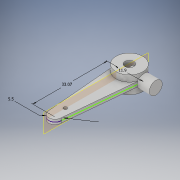
# Autodesk Inventor part: Nose Gear Steering Arm
Saved by Autodesk Inventor 2018 (Build 220112000, 112)
## iProperties
Created: 2018-08-04
Part Number: Nose Gear Steering Arm
Material: Generic
Document SubType Name: Modeling
Designer: Michael Gunderman
Density: 3.52387 g/cm^3
Appearance: Default
Mass: 5 g
Surface Area: 12.8518 cm^2
Volume: 1.41889 cm^3
Author: Michael Gunderman
Autodesk Inventor part; units mm, degrees
ref_plane "YZ Plane" through (0, 0, 0) normal (1, 0, 0) x (0, 1, 0)
ref_plane "XZ Plane" through (0, 0, 0) normal (0, 1, 0) x (-1, 0, 0)
ref_plane "XY Plane" through (0, 0, 0) normal (0, 0, 1) x (1, 0, 0)
sketch "Sketch1" plane through (0, 0, 0) normal (0, 1, 0) x (-1, 0, 0)
  circle A0 centre (0, 0) radius 5.95
  line L0 (0, 0) -> (0, 33.07)
  circle A1 centre (0, 33.07) radius 2.75
  line L1 (5.4153, 2.4652) -> (2.7393, 33.3118)
  line L2 (-5.8278, 1.1997) -> (-2.7497, 33.029)
  dimension "d0" = 11.9
  dimension "d1" = 5.5
  dimension "d2" = 33.07
  constraints: 6 end point, 4 point on circle, 2 centre point, 2 coincident, 1 vertical
  measures "d0" diameter of A0
  measures "d1" diameter of A1
  measures "d2" distance of L0.start L0.end
extrude "Extrusion1" add sketch "Sketch1" along normal mid plane 7.63 contours A0
extrude "Extrusion2" add sketch "Sketch1" along normal mid plane 2.1 contours A0 L0 A1 L1 | L2 A1 L0 A0 | A1
sketch "Sketch2" plane through (0, 1.05, 0) normal (0, 1, 0) x (1, 0, 0)
  arc A0 (-2.7393, -33.3118) -> (2.7497, -33.029) centre (0, -33.07) ccw construction
  line L0 (0, -35.82) -> (0, -28.45) construction
  circle A1 centre (0, -28.45) radius 0.75
  point P0 (0, 0)
  dimension "d7" = 7.37
  dimension "d8" = 1.5
  constraints: 2 end point, 1 centre point, 1 coincident, 1 point on circle, 1 vertical
  measures "d7" distance of L0.start L0.end
  measures "d8" diameter of A1
extrude "Extrusion3" cut sketch "Sketch2" against normal blind 2.1
sketch "Sketch3" plane through (0, 3.815, 0) normal (0, 1, 0) x (1, 0, 0)
  circle A0 centre (0, 0) radius 2
  point P0 (0, 0)
  dimension "d11" = 4
  constraints: 1 centre point, 1 coincident
  measures "d11" diameter of A0
extrude "Extrusion4" cut sketch "Sketch3" against normal blind 50
ref_plane "Work Plane1" through (-0.1567, -1.05, 63.0829) normal (0.9999878, 0, 0.004937) x (0, 1, 0)
sketch "Sketch4" plane through (-0.1567, -1.05, 63.0829) normal (0.9999878, 0, 0.004937) x (0, 1, 0)
  circle A0 centre (1.05, -63.6808) radius 2.85
  point P0 (1.05, -63.0829)
  dimension "d14" = 5.7
  constraints: 1 centre point
  measures "d14" diameter of A0
extrude "Extrusion5" add sketch "Sketch4" along normal blind 11
body "Solid1"
